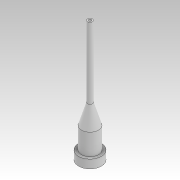
# Autodesk Inventor part: 14 Gauge Needle
Saved by Autodesk Inventor 2020 (Build 240168000, 168)
## iProperties
Created: 2021-09-12
Part Number: 14 Gauge Needle
Material: Generic
Document SubType Name: Modeling
Designer: DDeGo
Density: 1 g/cm^3
Appearance: Default
Author: DDeGo
Autodesk Inventor part; units mm, degrees
ref_plane "YZ Plane" through (0, 0, 0) normal (1, 0, 0) x (0, 1, 0)
ref_plane "XZ Plane" through (0, 0, 0) normal (0, 1, 0) x (-1, 0, 0)
ref_plane "XY Plane" through (0, 0, 0) normal (0, 0, 1) x (1, 0, 0)
sketch "Sketch1" plane through (0, 0, 0) normal (0, 0, 1) x (1, 0, 0)
  line L0 (0, 42.5) -> (0, 0) construction
  line L1 (0, 0) -> (0.5, 0) construction
  line L2 (4, 0) -> (4, 3)
  line L3 (4, 3) -> (3, 3)
  line L4 (3, 3) -> (3, 10.5)
  line L5 (3, 10.5) -> (0.9, 17.5)
  line L6 (0.9, 17.5) -> (0.9, 42.5)
  line L7 (0.9, 42.5) -> (0.5, 42.5)
  line L8 (0.5, 42.5) -> (0.5, 0)
  line L9 (0, 42.5) -> (0.5, 42.5) construction
  line L10 (0.5, 0) -> (4, 0)
  dimension "d0" = 0.5
  dimension "d1" = 0.9
  dimension "d2" = 25
  dimension "d3" = 3
  dimension "d4" = 4
  dimension "d5" = 3
  dimension "d6" = 7.5
  dimension "d7" = 17.5
  constraints: 22 end point, 10 perpendicular, 1 parallel, 1 vertical
  measures "d0" distance between parallel lines of L0 L8
  measures "d1" distance between parallel lines of L0 L6
  measures "d2" distance of L5.end L6.end
  measures "d3" distance of L2.start L2.end
  measures "d4" distance between parallel lines of L0 L2
  measures "d5" distance between parallel lines of L0 L4
  measures "d6" distance of L3.end L4.end
  measures "d7" distance from line of L10 L5.end
revolve "Revolution1" add sketch "Sketch1" angle 360 about axis through (0, 42.5, 0) along (0, -1, 0)
body "Solid1"
